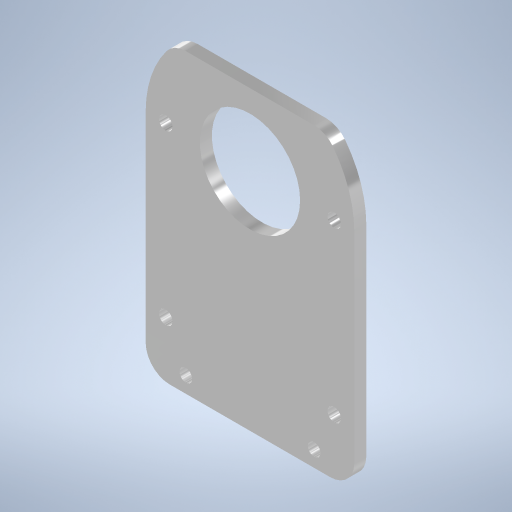
# Autodesk Inventor part: arm
Saved by Autodesk Inventor 2024.1 (Build 281209000, 209)
## iProperties
Created: 2024-02-14
Part Number: arm
Material: アルミニウム 6061
Document SubType Name: Sheet Metal
Designer: hibik
Density: 2.7 g/cm^3
Appearance: アルミニウム - フラット
Sheet Metal Rule: Default
Author: hibik
Autodesk Inventor part; units mm, degrees
ref_plane "YZ Plane" through (0, 0, 0) normal (1, 0, 0) x (0, 1, 0)
ref_plane "XZ Plane" through (0, 0, 0) normal (0, 1, 0) x (-1, 0, 0)
ref_plane "XY Plane" through (0, 0, 0) normal (0, 0, 1) x (1, 0, 0)
sketch "スケッチ2" plane through (0, 0, 0) normal (0, 0, 1) x (1, 0, 0)
  line L0 (0, 0) -> (26, 0)
  line L1 (26, 0) -> (26, 33)
  line L2 (26, 33) -> (0, 33)
  line L3 (0, 33) -> (0, 0)
  line L4 (0, 0) -> (26, 0)
  line L5 (26, 0) -> (26, 24)
  line L6 (26, 24) -> (0, 24) construction
  line L7 (0, 24) -> (0, 0)
  circle A0 centre (13, 24) radius 13
  circle A1 centre (13, 24) radius 6.25
  line L8 (26, 0) -> (0, 0)
  line L9 (0, 0) -> (0, -4)
  line L10 (0, -4) -> (26, -4)
  line L11 (26, -4) -> (26, 0)
  circle A2 centre (21, -2) radius 0.8
  circle A3 centre (5, -2) radius 0.8
  point P0 (22.3808, 33)
  point P1 (3.6192, 33)
  point P2 (26, -2)
  dimension "d0" = 26
  dimension "d1" = 33
  dimension "d2" = 24
  dimension "d3" = 12.5
  dimension "d8" = 4
  dimension "d9" = 1.6
  dimension "d10" = 1.6
  dimension "d12" = 5
  dimension "d13" = 5
  constraints: 24 end point, 6 parallel, 3 centre point, 3 horizontal, 3 perpendicular, 2 horizontal alignment, 2 midpoint, 1 coincident, 1 collinear, 1 point on line, 3 other
  measures "d0" distance of L1.end L2.end
  measures "d1" distance of L2.end L0.start
  measures "d2" distance between parallel lines of L0 L6
  measures "d3" diameter of A1
  measures "d8" distance of L8.end L9.end
  measures "d9" diameter of A2
  measures "d10" diameter of A3
  measures "d12" distance from line of L11 A2.centre
  measures "d13" distance from line of L9 A3.centre
extrude "押し出し1" add sketch "スケッチ2" along normal blind 1.5 contours L3 A0 L1 L0 | L0 L11 L10 L9 | A0 L2 picked at (12.7489, 32.0681)
sketch "スケッチ3" plane through (0, 0, 0) normal (0, 0, -1) x (-1, 0, 0)
  circle A0 centre (-2.5, 24) radius 0.85 projected
  circle A1 centre (-23.5, 24) radius 0.85 projected
  circle A2 centre (-23.5, 3) radius 0.85 projected
  circle A3 centre (-2.5, 3) radius 0.85 projected
  point P0 (0, 0)
extrude "押し出し2" cut sketch "スケッチ3" against normal through all
fillet "フィレット1" radius 3 4 edges at (22.3808, 33, 0.75) (3.6192, 33, 0.75) (26, -4, 0.75) (0, -4, 0.75)
equation "\"d13\" = d12"
equation "\"BendRadius\" = Thickness"
equation "\"BendReliefWidth\" = Thickness"
equation "\"BendReliefDepth\" = 0.5 * Thickness"
equation "\"CornerReliefSize\" = 4 * Thickness"
equation "\"MinimumRemnant\" = 2 * Thickness"
equation "\"TransitionRadius\" = BendRadius"
equation "\"JacobiRadiusSize\" = BendRadius"
equation "\"GapSize\" = Thickness"
equation "\"Thickness\" = 3.048"
